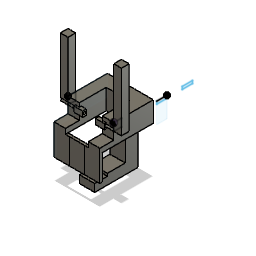
Pied rond piezo anna v5 v3 (Autodesk Fusion 360 archive; units mm, degrees)
design "levierFinal"
Autodesk Fusion 360 part; units mm, degrees
sketch "Sketch1" plane through (0, 0, 0) normal (0, 1, 0) x (1, 0, 0)
  line L0 (0, 0) -> (5, 0)
  line L1 (5, 0) -> (5, 5)
  line L2 (5, 5) -> (0, 5)
  line L3 (0, 5) -> (0, 0)
  line L4 (15, 0) -> (20, 0)
  line L5 (20, 0) -> (20, 5)
  line L6 (20, 5) -> (15, 5)
  line L7 (15, 5) -> (15, 0)
  line L8 (0, 5) -> (5, 0)
  line L9 (5, 5) -> (0, 0)
  circle A0 centre (2.5, 2.5) radius 1.25
  line L10 (15, 5) -> (20, 0)
  line L11 (20, 5) -> (15, 0)
  circle A1 centre (17.5, 2.5) radius 1.25
  line L12 (30, 7) -> (40, 7)
  line L13 (40, 7) -> (40, 0)
  line L14 (40, 0) -> (30, 0)
  line L15 (30, 0) -> (30, 7)
  line L16 (30, -3) -> (46, -3)
  line L17 (46, -3) -> (46, -9)
  line L18 (46, -9) -> (30, -9)
  line L19 (30, -9) -> (30, -3)
  line L20 (40, -3) -> (40, -9)
  dimension "d1" = 5
  dimension "d2" = 5
  dimension "d3" = 5
  dimension "d4" = 5
  dimension "d5" = 2.5
  dimension "d6" = 2.5
  dimension "d7" = 10
  dimension "d8" = 7
  dimension "d35" = 16
  dimension "d36" = 6
  dimension "d43" = 6
  constraint horizontal L0
  constraint vertical L1
  constraint horizontal L2
  constraint vertical L3
  constraint coincident L0.start L3.end
  constraint horizontal L4
  constraint vertical L5
  constraint horizontal L6
  constraint vertical L7
  constraint midpoint L9 A0.centre
  constraint midpoint L11 A1.centre
  constraint horizontal L12
  constraint vertical L13
  constraint horizontal L14
  constraint vertical L15
  constraint horizontal L16
  constraint vertical L17
  constraint horizontal L18
  constraint vertical L19
  constraint coincident L16 L20.start
  constraint coincident L18 L20.end
  constraint perpendicular L18 L20
  measures "d1" distance of L0.start L0.end
  measures "d2" distance of L0.start L2.end
  measures "d3" distance of L4.start L4.end
  measures "d4" distance of L4.start L6.end
  measures "d5" diameter of A0
  measures "d6" diameter of A1
  measures "d7" distance of L12.start L12.end
  measures "d8" distance of L12.start L14.end
  measures "d35" distance of L16.start L16.end
  measures "d36" distance of L16.start L18.end
  measures "d43" distance of L17 L20
extrude "Extrude1" add sketch "Sketch1" along normal blind 7 contours L12 L13 L14 L15 makes body 1
extrude "Extrude2" add sketch "Sketch1" along normal blind 4 separate body contours L0 L8 L9 A0 | L3 L8 L9 A0 | L1 L8 L9 A0 | L2 L8 L9 A0 makes body 2
extrude "Extrude3" add sketch "Sketch1" along normal blind 4 separate body contours L4 L10 L11 A1 | L7 L10 L11 A1 | L5 L10 L11 A1 | L6 L10 L11 A1 makes body 3
sketch "Sketch2" plane through (40, 0, 0) normal (1, 0, 0) x (0, 0, -1)
  line L0 (0, 0) -> (7, 0)
  line L1 (7, 0) -> (7, 7)
  line L2 (7, 7) -> (0, 7)
  line L3 (0, 7) -> (0, 0)
  line L4 (2.5, 2.5) -> (4.5, 2.5)
  line L5 (4.5, 2.5) -> (4.5, 4.5)
  line L6 (4.5, 4.5) -> (2.5, 4.5)
  line L7 (2.5, 4.5) -> (2.5, 2.5)
  dimension "d15" = -2.5
extrude "Extrude4" add sketch "Sketch2" along normal blind 10 contours L4 L5 L6 L7 bodies 1
sketch "Sketch3" plane through (50, 0, 0) normal (1, 0, 0) x (0, 0, -1)
  line L0 (2.5, 4.5) -> (2.5, 2.5)
  line L1 (2.5, 2.5) -> (4.5, 2.5)
  line L2 (4.5, 2.5) -> (4.5, 4.5)
  line L3 (4.5, 4.5) -> (2.5, 4.5)
  line L4 (-2.504, 4.5) -> (9.496, 4.5)
  line L5 (9.496, 4.5) -> (9.496, 2.5)
  line L6 (9.496, 2.5) -> (-2.504, 2.5)
  line L7 (-2.504, 2.5) -> (-2.504, 4.5)
  dimension "d18" = 12
  dimension "d19" = 2
  constraint horizontal L4
  constraint vertical L5
  constraint horizontal L6
  constraint vertical L7
  measures "d18" distance of L4.start L4.end
  measures "d19" distance of L4.start L6.end
extrude "Extrude5" add sketch "Sketch3" along normal blind 5 bodies 1
sketch "Sketch4" plane through (0, 0, -2.5) normal (0, 0, 1) x (1, 0, 0)
  line L0 (40, 4.5) -> (40, 2.5)
  line L1 (40, 2.5) -> (50, 2.5)
  line L2 (50, 2.5) -> (50, 4.5)
  line L3 (50, 4.5) -> (40, 4.5)
  circle A0 centre (42, 3.5) radius 0.5
  circle A1 centre (45, 3.5) radius 0.5
  circle A2 centre (48, 3.5) radius 0.5
extrude "Extrude6" cut sketch "Sketch4" against normal blind 2 contours A0 bodies 1
extrude "Extrude7" cut sketch "Sketch4" against normal blind 2 contours A1 bodies 1
extrude "Extrude8" cut sketch "Sketch4" against normal blind 2 contours A2 bodies 1
move_face "OffsetFaces1" offset -1.2 1 faces at (36.6667, 4.6667, 0) on bodies 1
move_face "OffsetFaces2" offset -1.2 1 faces at (33.3333, 4.6667, -7) on bodies 1
hole "Hole1" at (30, 3.5, -3.5) direction (1, 0, 0) diameter 3 depth 5 tip angle 180 bodies 1
move_face "OffsetFaces3" offset 3 1 faces at (5, 1.3333, -1.6667) on bodies 2
move_face "OffsetFaces4" offset 3 1 faces at (20, 1.3333, -1.6667) on bodies 3
extrude "Extrude10" add sketch "Sketch1" along normal blind 26 separate body contours L16 L17 L18 L20 makes body 4
extrude "Extrude11" add sketch "Sketch1" along normal blind 3 contours L16 L18 L19 L20 bodies 4
move_body "Move1" bodies 4 to x (0, -1, 0) y (1, 0, 0) z (0, 0, 1) at (30, 46, 0)
move_body "Move2" bodies 3 to x (1, 0, 0) y (0, 1, 0) z (0, 0, 1) at (33.8341, 0, 15.3688)
sketch "Sketch5" plane through (0, 0, 9) normal (0, 0, 1) x (1, 0, 0)
  line L0 (30, 16) -> (30, 0)
  line L1 (30, 0) -> (56, 0)
  line L2 (56, 0) -> (56, 6)
  line L3 (56, 6) -> (33, 6)
  line L4 (33, 6) -> (33, 16)
  line L5 (33, 16) -> (30, 16)
  line L6 (56, 6) -> (48, 6)
  line L7 (48, 6) -> (48, 0)
  line L8 (48, 0) -> (56, 0)
  line L9 (56, 0) -> (56, 6)
  dimension "d44" = 8
  constraint horizontal L6
  constraint vertical L7
  constraint horizontal L8
  constraint vertical L9
  constraint coincident L1 L7.end
  constraint coincident L2.end L3.start
  measures "d44" distance of L2.end L6.end
move_body "Move3" bodies 3 to x (1, 0, 0) y (0, 1, 0) z (0, 0, 1) at (-16.0824, 0, 6.7571)
extrude "Extrude12" add sketch "Sketch5" along normal blind 5 contours L1 L2 L3 L6 L7 L8 L9 bodies 4
move_body "Move4" bodies 1 to x (1, 0, 0) y (0, 1, 0) z (0, 0, 1) at (0, 0, 41.2945)
sketch "Sketch6" plane through (0, 0, 3) normal (0, 0, -1) x (-1, 0, 0)
  line L0 (-30, 0) -> (-30, 16)
  line L1 (-30, 16) -> (-33, 16)
  line L2 (-33, 16) -> (-33, 6)
  line L3 (-33, 6) -> (-56, 6)
  line L4 (-56, 6) -> (-56, 0)
  line L5 (-56, 0) -> (-30, 0)
  line L6 (-56, 6) -> (-48, 6)
  line L7 (-48, 6) -> (-48, 0)
  line L8 (-48, 0) -> (-56, 0)
  line L9 (-56, 0) -> (-56, 6)
  dimension "d47" = 8
  constraint horizontal L6
  constraint vertical L7
  constraint horizontal L8
  constraint vertical L9
  constraint coincident L5 L7.end
  constraint coincident L3.end L4.start
  measures "d47" distance of L3.end L6.end
extrude "Extrude13" add sketch "Sketch6" along normal blind 5 contours L3 L4 L5 L6 L7 L8 L9 bodies 4
sketch "Sketch7" plane through (33, 0, 0) normal (1, 0, 0) x (0, 0, -1)
  line L0 (-3, 6) -> (-3, 16)
  line L1 (-3, 16) -> (-9, 16)
  line L2 (-9, 16) -> (-9, 6)
  line L3 (-9, 6) -> (-3, 6)
extrude "Extrude14" add 1 faces at (31, 16, 7) along direction (0, 1, 0) blind 4 on bodies 4 bodies 4
sketch "Sketch8" plane through (33, 0, 0) normal (1, 0, 0) x (0, 0, -1)
  line L0 (-3, 6) -> (-3, 20)
  line L1 (-3, 20) -> (-9, 20)
  line L2 (-9, 20) -> (-9, 6)
  line L3 (-9, 6) -> (-3, 6)
  line L4 (-9, 20) -> (-3, 20)
  line L5 (-3, 20) -> (-3, 15)
  line L6 (-3, 15) -> (-9, 15)
  line L7 (-9, 15) -> (-9, 20)
  dimension "d52" = 5
  constraint horizontal L4
  constraint vertical L5
  constraint horizontal L6
  constraint vertical L7
  constraint coincident L0 L5.end
  constraint coincident L1.end L2.start
  measures "d52" distance of L1.end L6.end
extrude "Extrude15" add sketch "Sketch8" along normal blind 1 contours L0 L2 L3 L6 bodies 4
sketch "Sketch9" plane through (0, 6, 0) normal (0, 1, 0) x (-1, 0, 0)
  line L0 (-34, 3) -> (-34, 9)
  line L1 (-34, 9) -> (-48, 9)
  line L2 (-48, 9) -> (-48, 14)
  line L3 (-48, 14) -> (-56, 14)
  line L4 (-56, 14) -> (-56, -2)
  line L5 (-56, -2) -> (-48, -2)
  line L6 (-48, -2) -> (-48, 3)
  line L7 (-48, 3) -> (-34, 3)
  line L8 (-48, 9) -> (-56, 9)
  line L9 (-56, 9) -> (-56, 14)
  line L10 (-56, 14) -> (-48, 14)
  line L11 (-48, 14) -> (-48, 9)
  line L12 (-56, -2) -> (-48, -2)
  line L13 (-48, -2) -> (-48, 3)
  line L14 (-48, 3) -> (-56, 3)
  line L15 (-56, 3) -> (-56, -2)
  constraint horizontal L8
  constraint vertical L9
  constraint horizontal L10
  constraint vertical L11
  constraint coincident L3.end L4.start
  constraint coincident L1.end L2.start
  constraint horizontal L12
  constraint vertical L13
  constraint horizontal L14
  constraint vertical L15
  constraint coincident L6.end L7.start
  constraint coincident L4.end L5.start
extrude "Extrude16" add sketch "Sketch9" along normal blind 10 contours L4 L5 L6 L12 L13 L14 L15 bodies 4
extrude "Extrude17" add sketch "Sketch9" along normal blind 10 contours L2 L3 L4 L8 L9 L10 L11 bodies 4
move_body "Move5" bodies 3 to x (-1, 0, 0) y (0, 0, 1) z (0, 1, 0) at (65.5036, -17.126, 17.126)
move_body "Align1" bodies 4 to x (1, 0, 0) y (0, 1, 0) z (0, 0, 1) at (0, -16, 0)
move_body "Align2" bodies 3 to x (1, 0, 0) y (0, 1, 0) z (0, 0, 1) at (23.2482, 0, -8.126)
move_body "Move6" bodies 2 to x (-1, 0, 0) y (0, 0, 1) z (0, 1, 0) at (0, 5, -5)
move_body "Align3" bodies 2 to x (1, 0, 0) y (0, 1, 0) z (0, 0, 1) at (48, 0, 4)
move_body "Align4" bodies 2 to x (1, 0, 0) y (0, 1, 0) z (0, 0, 1) at (8, 0, 0)
sketch "Sketch10" plane through (0, 5, 0) normal (0, 1, 0) x (-1, 0, 0)
  line L0 (-56, 9) -> (-48, 9)
  line L1 (-48, 9) -> (-48, 13)
  line L2 (-48, 13) -> (-56, 13)
  line L3 (-56, 13) -> (-56, 9)
  line L4 (-48, 9) -> (-50, 9)
  line L5 (-50, 9) -> (-50, 13)
  line L6 (-50, 13) -> (-48, 13)
  line L7 (-48, 13) -> (-48, 9)
  dimension "d59" = 2
  constraint horizontal L4
  constraint vertical L5
  constraint horizontal L6
  constraint vertical L7
  constraint coincident L0.end L1.start
  measures "d59" distance of L0.end L4.end
sketch "Sketch11" plane through (0, 5, 0) normal (0, 1, 0) x (-1, 0, 0)
  line L0 (-56, -1) -> (-48, -1)
  line L1 (-48, -1) -> (-48, 3)
  line L2 (-48, 3) -> (-56, 3)
  line L3 (-56, 3) -> (-56, -1)
  line L4 (-48, -1) -> (-50, -1)
  line L5 (-50, -1) -> (-50, 3)
  line L6 (-50, 3) -> (-48, 3)
  line L7 (-48, 3) -> (-48, -1)
  dimension "d60" = 2
  constraint horizontal L4
  constraint vertical L5
  constraint horizontal L6
  constraint vertical L7
  constraint coincident L2 L5.end
  constraint coincident L0.end L1.start
  measures "d60" distance of L0.end L4.end
extrude "Extrude18" add sketch "Sketch11" along normal blind 3 contours L0 L1 L2 L4 L5 L6 L7 bodies 2
extrude "Extrude19" add sketch "Sketch10" along normal blind 3 contours L0 L1 L2 L4 L5 L6 L7 bodies 3
sketch "Sketch12" plane through (48, 0, 0) normal (-1, 0, 0) x (0, 0, 1)
  line L0 (9, 8) -> (9, 0)
  line L1 (9, 0) -> (13, 0)
  line L2 (13, 0) -> (13, 8)
  line L3 (13, 8) -> (9, 8)
  line L4 (3, 8) -> (-1, 8)
  line L5 (-1, 8) -> (-1, 7)
  line L6 (-1, 7) -> (3, 7)
  line L7 (3, 7) -> (3, 8)
  line L8 (9, 8) -> (13, 8)
  line L9 (13, 8) -> (13, 7)
  line L10 (13, 7) -> (9, 7)
  line L11 (9, 7) -> (9, 8)
  constraint horizontal L4
  constraint vertical L5
  constraint horizontal L6
  constraint vertical L7
  constraint horizontal L8
  constraint vertical L9
  constraint horizontal L10
  constraint vertical L11
  constraint coincident L0.start L3.end
extrude "Extrude20" add sketch "Sketch12" along normal blind 10 contours L4 L5 L6 L7 bodies 2
extrude "Extrude21" add sketch "Sketch12" along normal blind 10 contours L0 L2 L3 L8 L9 L10 L11 bodies 3
sketch "Sketch13" plane through (0, 0, 3) normal (0, 0, 1) x (1, 0, 0)
  circle A0 centre (53.5, 2.5) radius 1.25
  line L0 (56, 0) -> (56, 5)
  line L1 (56, 5) -> (50, 5)
  line L2 (50, 5) -> (50, 8)
  line L3 (50, 8) -> (38, 8)
  line L4 (38, 8) -> (38, 7)
  line L5 (38, 7) -> (48, 7)
  line L6 (48, 7) -> (48, 0)
  line L7 (48, 0) -> (56, 0)
  line L8 (48, 7) -> (50, 7)
  line L9 (50, 7) -> (50, 8)
  line L10 (50, 8) -> (48, 8)
  line L11 (48, 8) -> (48, 7)
  constraint horizontal L8
  constraint vertical L9
  constraint horizontal L10
  constraint vertical L11
  constraint coincident L2.end L3.start
  constraint coincident L5.end L6.start
extrude "Extrude22" add sketch "Sketch13" along normal blind 6 contours L3 L4 L5 L11 bodies 2 4 3
combine "Combine1" operation add target body 2 tool bodies 4
move_body "Move7" bodies 1 to x (1, 0, 0) y (0, 1, 0) z (0, 0, 1) at (-9.3863, 0, 0)
move_face "OffsetFaces5" offset 2 1 faces at (38.6667, -10, 7) on bodies 2
move_face "OffsetFaces6" offset -3 1 faces at (53.3333, -16, 7) on bodies 2
move_face "OffsetFaces7" offset 1 1 faces at (50.0833, 2.5, -1) on bodies 2
move_face "OffsetFaces8" offset 1 1 faces at (50.0833, 2.5, 13) on bodies 2
move_face "OffsetFaces9" offset 1 1 faces at (52.4073, -8.2396, 14) on bodies 2
move_face "OffsetFaces10" offset 1 1 faces at (52.4073, -8.2396, -2) on bodies 2
move_face "OffsetFaces11" offset -1 1 faces at (52.4073, -4.9062, 3) on bodies 2
move_face "OffsetFaces12" offset -1 1 faces at (52.4073, -4.9062, 9) on bodies 2
move_face "OffsetFaces13" offset -0.5 1 faces at (52.4073, -4.9062, 10) on bodies 2
move_face "OffsetFaces14" offset -0.5 1 faces at (52.4073, -4.9062, 2) on bodies 2
sketch "Sketch14" plane through (0, 0, 15) normal (0, 0, 1) x (1, 0, 0)
  circle A0 centre (53.5, 2.5) radius 1.25
  line L0 (56, -13) -> (56, 5)
  line L1 (56, 5) -> (50, 5)
  line L2 (50, 5) -> (50, 8)
  line L3 (50, 8) -> (38, 8)
  line L4 (38, 8) -> (38, 7)
  line L5 (38, 7) -> (48, 7)
  line L6 (48, 7) -> (48, -13)
  line L7 (48, -13) -> (56, -13)
  line L8 (50, 5) -> (56, 5)
  line L9 (56, 5) -> (56, 2.5)
  line L10 (56, 2.5) -> (50, 2.5)
  line L11 (50, 2.5) -> (50, 5)
  constraint horizontal L8
  constraint vertical L9
  constraint horizontal L10
  constraint vertical L11
  constraint coincident L0 L9.end
  constraint coincident L1.end L2.start
extrude "Extrude23" cut sketch "Sketch14" against normal blind 4.5 contours A0 L0 L1 L8 L9 L10 L11 bodies 2
sketch "Sketch15" plane through (0, 0, 1.5) normal (0, 0, 1) x (1, 0, 0)
  line L0 (48, 7) -> (48, -8)
  line L1 (48, -8) -> (56, -8)
  line L2 (56, -8) -> (56, 5)
  line L3 (56, 5) -> (50, 5)
  line L4 (50, 5) -> (50, 8)
  line L5 (50, 8) -> (48, 8)
  line L6 (48, 8) -> (48, 7)
  circle A0 centre (53.5, 2.5) radius 1.25
  line L7 (50, 5) -> (56, 5)
  line L8 (56, 5) -> (56, 2.5)
  line L9 (56, 2.5) -> (50, 2.5)
  line L10 (50, 2.5) -> (50, 5)
  constraint horizontal L7
  constraint vertical L8
  constraint horizontal L9
  constraint vertical L10
  constraint coincident L2 L8.end
  constraint coincident L3.end L4.start
extrude "Extrude24" cut sketch "Sketch15" against normal blind 4.5 contours L2 L3 A0 L7 L8 L9 L10 bodies 2
move_face "OffsetFaces15" offset 0.85 1 faces at (54.0359, 1.3707, 0) on bodies 2
move_face "OffsetFaces16" offset 0.85 1 faces at (52.2562, 2.3755, 13.5) on bodies 2
delete_face "DeleteFace1" 1 faces at (22.2804, 3.7406, 39.2751) on bodies 1
extrude "Extrude25" cut 1 faces at (23.9471, 4.6667, 35.4945) along direction (0, 0, 1) blind 1.3 on bodies 1 bodies 1
extrude "Extrude26" cut 1 faces at (27.2804, 4.6667, 40.0945) along direction (0, 0, -1) blind 1.3 on bodies 1 bodies 1
sketch "Sketch16" plane through (0, 0, 38.7945) normal (0, 0, 1) x (1, 0, 0)
  circle A0 centre (38.6137, 3.5) radius 0.5
  circle A1 centre (35.6137, 3.5) radius 0.5
  circle A2 centre (32.6137, 3.5) radius 0.5
  line L0 (30.6137, 2.5) -> (40.6137, 2.5)
  line L1 (40.6137, 2.5) -> (40.6137, 4.5)
  line L2 (40.6137, 4.5) -> (30.6137, 4.5)
  line L3 (30.6137, 4.5) -> (30.6137, 7)
  line L4 (30.6137, 7) -> (20.6137, 7)
  line L5 (20.6137, 7) -> (20.6137, 0)
  line L6 (20.6137, 0) -> (30.6137, 0)
  line L7 (30.6137, 0) -> (30.6137, 2.5)
  line L8 (36.6137, 4.5) -> (34.6137, 4.5)
  line L9 (34.6137, 4.5) -> (34.6137, 2.5)
  line L10 (34.6137, 2.5) -> (36.6137, 2.5)
  line L11 (36.6137, 2.5) -> (36.6137, 4.5)
  dimension "d91" = 1
  dimension "d92" = 2
  constraint horizontal L8
  constraint vertical L9
  constraint horizontal L10
  constraint vertical L11
  constraint coincident L0 L9.end
  constraint coincident L2 L8.start
  measures "d91" distance of A1.centre L9
  measures "d92" distance of L8.start L8.end
move_face "OffsetFaces21" offset 0.997 1 faces at (38.8194, 3.9558, 37.4612) on bodies 1
move_face "OffsetFaces22" offset 0.668 1 faces at (32.8194, 3.9558, 37.4612) on bodies 1
move_face "OffsetFaces23" offset -1 1 faces at (20.6137, 2.3333, 38.1278) on bodies 1
sketch "Sketch18" plane through (0, 2.5, 0) normal (0, 1, 0) x (-1, 0, 0)
  line L0 (-50, 15) -> (-53.1, 15)
  line L1 (-53.1, 15) -> (-53.1, 10.5)
  line L2 (-53.1, 10.5) -> (-50, 10.5)
  line L3 (-50, 10.5) -> (-50, 15)
  line L4 (-52.3705, 10.5) -> (-54.5, 10.5)
  line L5 (-54.5, 10.5) -> (-54.5, 12)
  line L6 (-54.5, 12) -> (-52.3705, 12)
  line L7 (-52.3705, 12) -> (-52.3705, 10.5)
  constraint horizontal L4
  constraint vertical L5
  constraint horizontal L6
  constraint vertical L7
  constraint coincident L2 L4.start
extrude "Extrude29" add sketch "Sketch18" along normal blind 0.4 contours L1 L2 L4 L6 L7 | L1 L4 L5 L6 bodies 2
sketch "Sketch19" plane through (0, 0, 10.5) normal (0, 0, -1) x (-1, 0, 0)
  arc A0 (-53.9, 2.5) -> (-53.1, 2.5) centre (-53.5, 2.5) ccw
  line L0 (-53.9, 2.5) -> (-53.1, 2.5)
  line L1 (-52.3705, 2.5) -> (-52.3705, 2.9)
  line L2 (-52.3705, 2.9) -> (-54.5, 2.9)
  line L3 (-54.5, 2.9) -> (-54.5, 2.5)
  line L4 (-54.5, 2.5) -> (-56, 2.5)
  line L5 (-56, 2.5) -> (-56, -8)
  line L6 (-56, -8) -> (-48, -8)
  line L7 (-48, -8) -> (-48, 7)
  line L8 (-48, 7) -> (-48, 8)
  line L9 (-48, 8) -> (-50, 8)
  line L10 (-50, 8) -> (-50, 2.5)
  line L11 (-50, 2.5) -> (-52.3705, 2.5)
  circle A1 centre (-53.5, 2.5) radius 0.4
  constraint concentric A0 A1
  constraint coincident A0.end A1
extrude "Extrude30" add 1 faces at (53.7902, 2.9, 11.5) along direction (0, 1, 0) blind 0.1 on bodies 2 bodies 2
extrude "Extrude31" cut sketch "Sketch19" against normal blind 1.687 contours L0 A1 bodies 2
sketch "Sketch20" plane through (0, 0, 10.5) normal (0, 0, -1) x (-1, 0, 0)
  line L0 (-52.3705, 2.5) -> (-52.3705, 3)
  line L1 (-52.3705, 3) -> (-54.5, 3)
  line L2 (-54.5, 3) -> (-54.5, 2.5)
  line L3 (-54.5, 2.5) -> (-56, 2.5)
  line L4 (-56, 2.5) -> (-56, -8)
  line L5 (-56, -8) -> (-48, -8)
  line L6 (-48, -8) -> (-48, 7)
  line L7 (-48, 7) -> (-48, 8)
  line L8 (-48, 8) -> (-50, 8)
  line L9 (-50, 8) -> (-50, 2.5)
  line L10 (-50, 2.5) -> (-52.3705, 2.5)
  circle A0 centre (-53.5, 2.5) radius 0.4
  line L11 (-54.5, 2.5) -> (-53.9, 2.5)
  line L12 (-53.1, 2.5) -> (-52.3705, 2.5)
  line L13 (-54.5, 2.5) -> (-52.3705, 2.5)
  line L14 (-52.3705, 2.5) -> (-52.3705, 1.7972)
  line L15 (-52.3705, 1.7972) -> (-54.5, 1.7972)
  line L16 (-54.5, 1.7972) -> (-54.5, 2.5)
  point P0 (-53.1, 2.5)
  constraint coincident L2.end L3.start
  constraint coincident A0 L11.end
  constraint perpendicular L2 L11
  constraint coincident P0 L12.start
  constraint coincident L0.start L10.end
  constraint horizontal L13
  constraint vertical L14
  constraint horizontal L15
  constraint vertical L16
extrude "Extrude32" add sketch "Sketch20" along normal blind 2 contours L0 L1 L2 A0 L11 L12 L13 | A0 L11 L12 L13 L14 L15 L16 bodies 2
sketch "Sketch21" plane through (0, 2.5, 0) normal (0, 1, 0) x (-1, 0, 0)
  line L0 (-53.9, 1.5) -> (-56, 1.5)
  line L1 (-56, 1.5) -> (-56, -3)
  line L2 (-56, -3) -> (-53.9, -3)
  line L3 (-53.9, -3) -> (-53.9, 1.5)
  line L4 (-53.9, 1.5) -> (-54.5, 1.5)
  line L5 (-54.5, 1.5) -> (-54.5, 0)
  line L6 (-54.5, 0) -> (-53.9, 0)
  line L7 (-53.9, 0) -> (-53.9, 1.5)
  line L8 (-54.5, 0) -> (-52.37, 0)
  line L9 (-52.37, 0) -> (-52.37, 1.5)
  line L10 (-52.37, 1.5) -> (-54.5, 1.5)
  line L11 (-54.5, 1.5) -> (-54.5, 0)
  dimension "d114" = 0.6
  dimension "d115" = 1.5
  dimension "d116" = 2.13
  constraint horizontal L4
  constraint vertical L5
  constraint horizontal L6
  constraint vertical L7
  constraint coincident L0.start L3.end
  constraint horizontal L8
  constraint vertical L9
  constraint horizontal L10
  constraint vertical L11
  measures "d114" distance of L0.start L4.end
  measures "d115" distance of L0.start L6.end
  measures "d116" distance of L5.end L8.end
extrude "Extrude33" add sketch "Sketch21" along normal blind 0.5 contours L0 L3 L4 L5 L6 L7 L8 L10 L11 | L3 L7 L8 L9 L10 bodies 2
sketch "Sketch22" plane through (0, 0, 1.5) normal (0, 0, 1) x (1, 0, 0)
  line L0 (52.37, 2.5) -> (50, 2.5)
  line L1 (50, 2.5) -> (50, 8)
  line L2 (50, 8) -> (48, 8)
  line L3 (48, 8) -> (48, 7)
  line L4 (48, 7) -> (48, -8)
  line L5 (48, -8) -> (56, -8)
  line L6 (56, -8) -> (56, 2.5)
  line L7 (56, 2.5) -> (54.5, 2.5)
  line L8 (54.5, 2.5) -> (54.5, 3)
  line L9 (54.5, 3) -> (52.37, 3)
  line L10 (52.37, 3) -> (52.37, 2.5)
  line L11 (53.1, 2.5) -> (53.9, 2.5)
  arc A0 (53.1, 2.5) -> (53.9, 2.5) centre (53.5, 2.5) ccw
  circle A1 centre (53.5, 2.5) radius 0.4
  constraint concentric A0 A1
  constraint coincident L11.end A1
extrude "Extrude34" cut sketch "Sketch22" against normal blind 1.863 contours L11 A1 bodies 2
sketch "Sketch23" plane through (0, 0, 1.5) normal (0, 0, 1) x (1, 0, 0)
  circle A0 centre (53.5, 2.5) radius 0.4
  line L0 (52.37, 2.5) -> (50, 2.5)
  line L1 (50, 2.5) -> (50, 8)
  line L2 (50, 8) -> (48, 8)
  line L3 (48, 8) -> (48, 7)
  line L4 (48, 7) -> (48, -8)
  line L5 (48, -8) -> (56, -8)
  line L6 (56, -8) -> (56, 2.5)
  line L7 (56, 2.5) -> (54.5, 2.5)
  line L8 (54.5, 2.5) -> (54.5, 3)
  line L9 (54.5, 3) -> (52.37, 3)
  line L10 (52.37, 3) -> (52.37, 2.5)
  line L11 (54.5, 3) -> (52.37, 3)
  line L12 (52.37, 3) -> (52.37, 2)
  line L13 (52.37, 2) -> (54.5, 2)
  line L14 (54.5, 2) -> (54.5, 3)
  dimension "d121" = 1
  constraint horizontal L11
  constraint vertical L12
  constraint horizontal L13
  constraint vertical L14
  constraint coincident L8.end L9.start
  measures "d121" distance of L8.end L13.end
extrude "Extrude35" add sketch "Sketch23" along normal blind 2 contours L8 L9 L10 L11 L12 L13 L14 bodies 2
move_face "OffsetFaces24" offset 0.2 1 faces at (53.7902, 3, 10.8333) on bodies 2
move_face "OffsetFaces25" offset 0.2 1 faces at (53.79, 3, 1.1667) on bodies 2
move_face "OffsetFaces26" offset 0.2 1 faces at (53.08, 2, 2.1667) on bodies 2
move_face "OffsetFaces27" offset -0.1 1 faces at (53.102, 2.4602, 0.1667) on bodies 2
move_face "OffsetFaces28" offset -0.1 1 faces at (53.102, 2.4602, 11.8333) on bodies 2
delete_body "RemoveBody1" bodies 1
move_body "Move8" bodies 2 to x (0, 1, 0) y (0, 0, 1) z (1, 0, 0) at (4.4665, -65.6113, 8.6253)
move_body "Move9" bodies 2 to x (1, 0, 0) y (0, 1, 0) z (0, 0, 1) at (9.7685, 0, 0)
sketch "Sketch26" plane through (11.2351, 0, 0) normal (-1, 0, 0) x (0, 0, 1)
  line L0 (11.1253, -11.6113) -> (11.1253, -9.6113)
  line L1 (11.1253, -9.6113) -> (-4.3747, -9.6113)
  line L2 (-4.3747, -9.6113) -> (-4.3747, -17.6113)
  line L3 (-4.3747, -17.6113) -> (15.6253, -17.6113)
  line L4 (15.6253, -17.6113) -> (15.6253, -27.6113)
  line L5 (15.6253, -27.6113) -> (16.6253, -27.6113)
  line L6 (16.6253, -27.6113) -> (16.6253, -15.6113)
  line L7 (16.6253, -15.6113) -> (11.1253, -15.6113)
  line L8 (11.1253, -15.6113) -> (11.1253, -12.6113)
  arc A0 (11.1253, -11.6113) -> (11.1253, -12.6113) centre (11.1253, -12.1113) ccw
  line L9 (11.1253, -9.6113) -> (8.1253, -9.6113)
  line L10 (8.1253, -9.6113) -> (8.1253, -12.6113)
  line L11 (8.1253, -12.6113) -> (11.1253, -12.6113)
  line L12 (11.1253, -12.6113) -> (11.1253, -9.6113)
  line L13 (11.1253, -9.6113, -18) -> (8.1253, -9.6113, -18)
  line L14 (8.1253, -9.6113, -18) -> (8.1253, -12.6113, -18)
  line L15 (8.1253, -12.6113, -18) -> (11.1253, -12.6113, -18)
  line L16 (11.1253, -12.6113, -18) -> (11.1253, -9.6113, -18)
  point P0 (11.1253, -9.6113)
  dimension "d143" = 3
  dimension "d144" = 3
  dimension "d145" = 3
  dimension "d146" = 3
  constraint horizontal L9
  constraint vertical L10
  constraint horizontal L11
  constraint vertical L12
  constraint coincident P0 L0.end
  measures "d143" distance of P0 L9.end
  measures "d144" distance of P0 L8.end
  measures "d145" distance of P0 L9.end
  measures "d146" distance of P0 L8.end
extrude "Extrude40" add sketch "Sketch26" against normal blind 3 contours L13 L14 L15 L16 in plane through (29.2351, 0, 0) normal (-1, 0, 0) bodies 2
extrude "Extrude41" add sketch "Sketch26" along normal blind 3 contours L0 L1 A0 L9 L10 L11 L12 bodies 2
sketch "Sketch27" plane through (0, -9.6113, 0) normal (0, 1, 0) x (-1, 0, 0)
  line L0 (-8.2351, 11.1253) -> (-15.7351, 11.1253)
  line L1 (-15.7351, 11.1253) -> (-15.7351, 0.6253)
  line L2 (-15.7351, 0.6253) -> (-24.7351, 0.6253)
  line L3 (-24.7351, 0.6253) -> (-24.7351, 11.1253)
  line L4 (-24.7351, 11.1253) -> (-32.2351, 11.1253)
  line L5 (-32.2351, 11.1253) -> (-32.2351, 8.1253)
  line L6 (-32.2351, 8.1253) -> (-29.2351, 8.1253)
  line L7 (-29.2351, 8.1253) -> (-29.2351, -4.3747)
  line L8 (-29.2351, -4.3747) -> (-11.2351, -4.3747)
  line L9 (-11.2351, -4.3747) -> (-11.2351, 8.1253)
  line L10 (-11.2351, 8.1253) -> (-8.2351, 8.1253)
  line L11 (-8.2351, 8.1253) -> (-8.2351, 11.1253)
  line L12 (-8.2351, 11.1253) -> (-11.2351, 11.1253)
  line L13 (-11.2351, 11.1253) -> (-11.2351, 8.1253)
  line L14 (-11.2351, 8.1253) -> (-8.2351, 8.1253)
  line L15 (-8.2351, 8.1253) -> (-8.2351, 11.1253)
  line L16 (-32.2351, 11.1253) -> (-29.2351, 11.1253)
  line L17 (-29.2351, 11.1253) -> (-29.2351, 8.1253)
  line L18 (-29.2351, 8.1253) -> (-32.2351, 8.1253)
  line L19 (-32.2351, 8.1253) -> (-32.2351, 11.1253)
  constraint horizontal L12
  constraint vertical L13
  constraint horizontal L14
  constraint vertical L15
  constraint coincident L9.end L10.start
  constraint coincident L0.start L11.end
  constraint horizontal L16
  constraint vertical L17
  constraint horizontal L18
  constraint vertical L19
  constraint coincident L6.end L7.start
  constraint coincident L4.end L5.start
extrude "Extrude42" add sketch "Sketch27" along normal blind 20 contours L0 L10 L11 L12 L13 L14 L15 bodies 2
sketch "Sketch28" plane through (0, -9.6113, 0) normal (0, 1, 0) x (-1, 0, 0)
  line L0 (-11.2351, 8.1253) -> (-11.2351, 11.1253)
  line L1 (-11.2351, 11.1253) -> (-15.7351, 11.1253)
  line L2 (-15.7351, 11.1253) -> (-15.7351, 0.6253)
  line L3 (-15.7351, 0.6253) -> (-24.7351, 0.6253)
  line L4 (-24.7351, 0.6253) -> (-24.7351, 11.1253)
  line L5 (-24.7351, 11.1253) -> (-32.2351, 11.1253)
  line L6 (-32.2351, 11.1253) -> (-32.2351, 8.1253)
  line L7 (-32.2351, 8.1253) -> (-29.2351, 8.1253)
  line L8 (-29.2351, 8.1253) -> (-29.2351, -4.3747)
  line L9 (-29.2351, -4.3747) -> (-11.2351, -4.3747)
  line L10 (-11.2351, -4.3747) -> (-11.2351, 8.1253)
  line L11 (-32.2351, 11.1253) -> (-29.2351, 11.1253)
  line L12 (-29.2351, 11.1253) -> (-29.2351, 8.1253)
  line L13 (-29.2351, 8.1253) -> (-32.2351, 8.1253)
  line L14 (-32.2351, 8.1253) -> (-32.2351, 11.1253)
  constraint horizontal L11
  constraint vertical L12
  constraint horizontal L13
  constraint vertical L14
  constraint coincident L7.end L8.start
  constraint coincident L5.end L6.start
extrude "Extrude43" add sketch "Sketch28" along normal blind 20 contours L5 L6 L7 L11 L12 L13 L14 bodies 2
